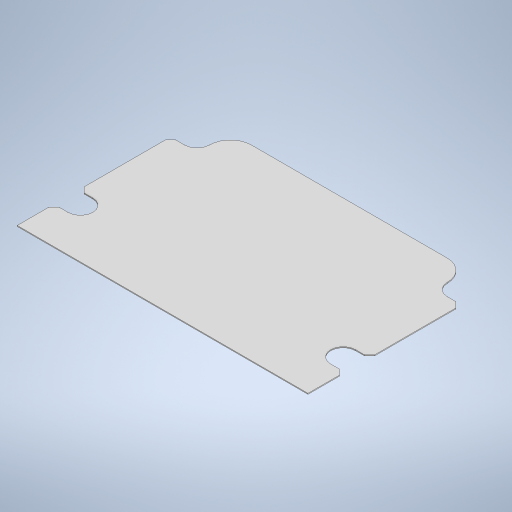
# Autodesk Inventor part: oddělovací plocha
Saved by Autodesk Inventor 2024 (Build 280153000, 153)
## iProperties
Created: 2023-09-06
Part Number: oddělovací plocha
Material: Všeobecné
Document SubType Name: Modeling
Designer: Simak
Density: 1 g/cm^3
Appearance: Výchozí
Author: Simak
Autodesk Inventor part; units mm, degrees
ref_plane "YZ Plane" through (0, 0, 0) normal (1, 0, 0) x (0, 1, 0)
ref_plane "XZ Plane" through (0, 0, 0) normal (0, 1, 0) x (-1, 0, 0)
ref_plane "Pracovní rovina16" through (0, 5, 0) normal (0, -1, 0) x (1, 0, 0)
sketch "Náčrt80" plane through (0, 5, 0) normal (0, -1, 0) x (1, 0, 0)
  circle A0 centre (-22, -24.1875) radius 1.85 projected
  circle A1 centre (22, -24.1875) radius 1.85 projected
  circle A2 centre (-42.25, -8.5) radius 1.85 projected
  circle A3 centre (-42.25, 29) radius 1.85 projected
  circle A4 centre (42.25, -8.5) radius 1.85 projected
  circle A5 centre (42.25, 29) radius 1.85 projected
  arc A6 (-38.75, -8.5) -> (-42.25, -5) centre (-42.25, -8.5) ccw projected
  line L0 (-45.25, -5) -> (-42.25, -5) projected
  line L1 (-47.25, -3) -> (-45.25, -5) projected
  line L2 (-47.25, 23.5) -> (-47.25, -3) projected
  line L3 (-45.25, 25.5) -> (-47.25, 23.5) projected
  line L4 (-42.25, 25.5) -> (-45.25, 25.5) projected
  arc A7 (-42.25, 25.5) -> (-42.25, 32.5) centre (-42.25, 29) ccw projected
  line L5 (-45.25, 32.5) -> (-42.25, 32.5) projected
  line L6 (-47.25, 34.5) -> (-45.25, 32.5) projected
  line L7 (-47.25, 45.3044) -> (-47.25, 34.5) projected
  line L8 (47.25, 45.3044) -> (-47.25, 45.3044) projected
  line L9 (47.25, 34.5) -> (47.25, 45.3044) projected
  line L10 (45.25, 32.5) -> (47.25, 34.5) projected
  line L11 (42.25, 32.5) -> (45.25, 32.5) projected
  arc A8 (42.25, 32.5) -> (42.25, 25.5) centre (42.25, 29) ccw projected
  line L12 (45.25, 25.5) -> (42.25, 25.5) projected
  line L13 (47.25, 23.5) -> (45.25, 25.5) projected
  line L14 (47.25, -3) -> (47.25, 23.5) projected
  line L15 (45.25, -5) -> (47.25, -3) projected
  line L16 (42.25, -5) -> (45.25, -5) projected
  arc A9 (42.25, -5) -> (38.75, -8.5) centre (42.25, -8.5) ccw projected
  arc A10 (31.5, -15.75) -> (38.75, -8.5) centre (31.5, -8.5) ccw projected
  line L17 (31.5, -15.75) -> (-31.5, -15.75) projected
  arc A11 (-38.75, -8.5) -> (-31.5, -15.75) centre (-31.5, -8.5) ccw projected
  line L18 (-5, -41.375) -> (-5, -35.875) projected
  arc A12 (5, -35.875) -> (-5, -35.875) centre (0, -35.875) ccw projected
  line L19 (5, -41.375) -> (5, -35.875) projected
  line L20 (5, -41.375) -> (-5, -41.375) projected
  arc A13 (-20.6747, -48.0519) -> (-23.3253, -48.0519) centre (-22, -44.8125) ccw projected
  line L21 (-0.0392, -48.0519) -> (-20.6747, -48.0519) projected
  line L22 (-2.825, -46.4435) -> (-0.0392, -48.0519) projected
  line L23 (-2.825, -43.1815) -> (-2.825, -46.4435) projected
  line L24 (0, -41.5505) -> (-2.825, -43.1815) projected
  line L25 (2.825, -43.1815) -> (0, -41.5505) projected
  line L26 (2.825, -46.4435) -> (2.825, -43.1815) projected
  line L27 (0.0392, -48.0519) -> (2.825, -46.4435) projected
  line L28 (20.6747, -48.0519) -> (0.0392, -48.0519) projected
  arc A14 (23.3253, -48.0519) -> (20.6747, -48.0519) centre (22, -44.8125) ccw projected
  line L29 (27, -48.0519) -> (23.3253, -48.0519) projected
  line L30 (27, -19.25) -> (27, -48.0519) projected
  line L31 (49.75, -19.25) -> (27, -19.25) projected
  line L32 (49.75, 48.4103) -> (49.75, -19.25) projected
  line L33 (-49.75, 48.4103) -> (49.75, 48.4103) projected
  line L34 (-49.75, -19.25) -> (-49.75, 48.4103) projected
  line L35 (-27, -19.25) -> (-49.75, -19.25) projected
  line L36 (-27, -48.0519) -> (-27, -19.25) projected
  line L37 (-23.3253, -48.0519) -> (-27, -48.0519) projected
  line L38 (-31.5, -15.25) -> (31.5, -15.25)
  arc A15 (31.5, -15.25) -> (38.25, -8.5) centre (31.5, -8.5) ccw
  arc A16 (42.25, -4.5) -> (38.25, -8.5) centre (42.25, -8.5) ccw
  line L39 (42.25, -4.5) -> (45.0429, -4.5)
  line L40 (45.0429, -4.5) -> (46.75, -2.7929)
  line L41 (46.75, -2.7929) -> (46.75, 23.2929)
  line L42 (46.75, 23.2929) -> (45.0429, 25)
  line L43 (45.0429, 25) -> (42.25, 25)
  arc A17 (42.25, 33) -> (42.25, 25) centre (42.25, 29) ccw
  line L44 (42.25, 33) -> (45.0429, 33)
  line L45 (45.0429, 33) -> (46.75, 34.7071)
  line L46 (46.75, 34.7071) -> (46.75, 44.8044)
  line L47 (46.75, 44.8044) -> (-46.75, 44.8044)
  line L48 (-46.75, 44.8044) -> (-46.75, 34.7071)
  line L49 (-46.75, 34.7071) -> (-45.0429, 33)
  line L50 (-45.0429, 33) -> (-42.25, 33)
  arc A18 (-42.25, 25) -> (-42.25, 33) centre (-42.25, 29) ccw
  line L51 (-42.25, 25) -> (-45.0429, 25)
  line L52 (-45.0429, 25) -> (-46.75, 23.2929)
  line L53 (-46.75, 23.2929) -> (-46.75, -2.7929)
  line L54 (-46.75, -2.7929) -> (-45.0429, -4.5)
  line L55 (-45.0429, -4.5) -> (-42.25, -4.5)
  arc A19 (-38.25, -8.5) -> (-42.25, -4.5) centre (-42.25, -8.5) ccw
  arc A20 (-38.25, -8.5) -> (-31.5, -15.25) centre (-31.5, -8.5) ccw
  point P0 (0, 0)
  dimension "d487" = 0.5
  constraints: 36 end point, 12 point on circle, 6 centre point, 23 other
  measures "d487" distance between parallel lines of L17 L38
extrude "Vysunutí84" add sketch "Náčrt80" against normal blind 0.3 contours A20 A19 L55 L54 L53 L52 L51 A18 L50 L49 L48 L47 L46 L45 L44 A17 L43 L42 L41 L40 L39 A16 A15 L38
